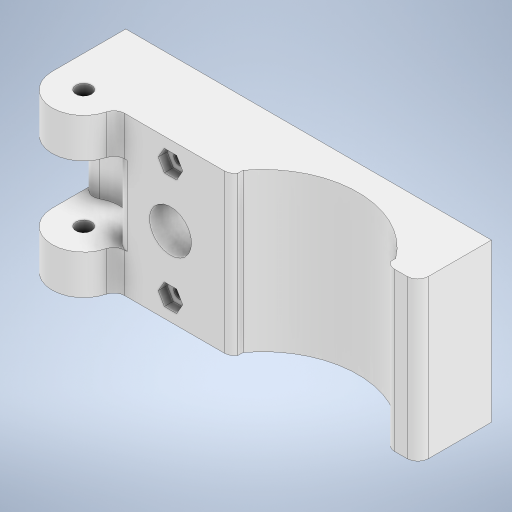
# Autodesk Inventor part: Bike_Mount_Right
Saved by Autodesk Inventor 2023 (Build 270158000, 158)
## iProperties
Created: 2023-01-23
Part Number: Bike_Mount_Right
Material: PC/ABS Plastic
Document SubType Name: Modeling
Designer: manny
Density: 0.357273 g/cm^3
Appearance: White
Author: manny
Autodesk Inventor part; units mm, degrees
ref_plane "YZ Plane" through (0, 0, 0) normal (1, 0, 0) x (0, 1, 0)
ref_plane "XZ Plane" through (0, 0, 0) normal (0, 1, 0) x (-1, 0, 0)
ref_plane "XY Plane" through (0, 0, 0) normal (0, 0, 1) x (1, 0, 0)
sketch "Sketch2" plane through (0, 0, 0) normal (0, 1, 0) x (-1, 0, 0)
  arc A0 (2, 14) -> (0, 12) centre (2, 12) ccw
  arc A1 (6.0742, 13.1179) -> (35.0957, 13.1179) centre (20.5849, 22.9) ccw
  line L0 (36.754, 14) -> (55.754, 14)
  arc A2 (69.5, 14) -> (57.6905, 15.5) centre (63.5, 14) ccw
  circle A3 centre (63.5, 14) radius 1.5
  arc A4 (55.754, 14) -> (57.6905, 15.5) centre (55.754, 16) ccw
  arc A5 (36.754, 14) -> (35.0957, 13.1179) centre (36.754, 12) ccw
  arc A6 (6.0742, 13.1179) -> (4.4158, 14) centre (4.4158, 12) ccw
  arc A7 (57.3882, 12.2181) -> (55.2287, 14) centre (55.2287, 11.8005) ccw
  line L1 (0, 12) -> (0, 0)
  line L2 (0, 0) -> (69.5, 0)
  line L3 (69.5, 14) -> (69.5, 0)
  arc A8 (57.3882, 12.2181) -> (69.5, 11.7415) centre (63.5, 13.4) ccw
  line L4 (4.4158, 14) -> (2, 14)
  point P0 (0, 0)
  point P1 (20.5849, 5.4)
  dimension "d3" = 2
  dimension "d17" = 3
  dimension "d18" = 2
  dimension "d137" = 2.1995
  dimension "d140" = 12
  dimension "d141" = 69.5
  dimension "d142" = 14
  dimension "d143" = 6
  dimension "d144" = 17.5
  dimension "d145" = 19
  dimension "d146" = 5.4
  dimension "d147" = 6.225
  dimension "d148" = 13.4
  constraints: 18 point on circle, 11 tangent, 10 end point, 9 centre point, 5 point on line, 3 horizontal, 2 vertical, 1 coincident, 1 equal radius, 1 horizontal alignment, 1 vertical alignment
  measures "d3" radius of A0
  measures "d17" diameter of A3
  measures "d18" radius of A4
  measures "d137" radius of A7
  measures "d140" distance from line of L2 A0.centre
  measures "d141" distance of L1.end L2.end
  measures "d142" distance of L3.start L2.end
  measures "d143" radius of A2
  measures "d144" radius of A1
  measures "d145" distance of L0.start L0.end
  measures "d146" distance from line of L2 point (20.585, 5.4)
  measures "d147" radius of A8
  measures "d148" vertical distance of point (0, 0) A8.centre
extrude "Extrusion1" add sketch "Sketch2" along normal mid plane 30
extrude "Extrusion2" cut sketch "Sketch2" along normal mid plane 15 contours A8 A7 L0 A4 A2 L3
sketch "Sketch7" plane through (0, -15, 0) normal (0, -1, 0) x (1, 0, 0)
  arc A0 (-4.4158, 14) -> (-6.0742, 13.1179) centre (-4.4158, 12) ccw projected
  line L0 (-6.0742, 13.1179) -> (-6.0742, 12.1179)
  arc A1 (-35.0957, 13.1179) -> (-6.0742, 13.1179) centre (-20.5849, 22.9) ccw projected
  line L1 (-35.0957, 13.1179) -> (-35.0957, 12.1179)
  arc A2 (-35.0957, 12.1179) -> (-6.0742, 12.1179) centre (-20.5849, 22.8831) ccw
  point P0 (0, 0)
  point P1 (-6.3389, 0)
  dimension "d59" = 1
  dimension "d60" = 1
  constraints: 4 end point, 2 point on circle, 2 vertical, 1 centre point
  measures "d59" distance of L0.start L0.end
  measures "d60" distance of L1.start L1.end
extrude "Extrusion10" cut sketch "Sketch7" against normal up to next
fillet "Fillet4" radius 2 1 edges at (-69.5, 0, 11.7415)
sketch "Sketch13" plane through (-55.754, -15, 14) normal (0, 0, 1) x (1, 0, 0)
  circle A0 centre (8.754, 15) radius 4
  line L0 (55.754, 0) -> (55.754, 30) projected
  line L1 (14.254, 18.1754) -> (14.254, 11.8246)
  line L2 (14.254, 11.8246) -> (8.754, 8.6491)
  line L3 (8.754, 8.6491) -> (3.254, 11.8246)
  line L4 (3.254, 11.8246) -> (3.254, 18.1754)
  line L5 (3.254, 18.1754) -> (8.754, 21.3509)
  line L6 (8.754, 21.3509) -> (14.254, 18.1754)
  line L7 (19, 0) -> (0, 0) projected
  circle A1 centre (8.754, 26) radius 1.1
  line L8 (8.754, 15) -> (25.6273, 15) construction
  line L9 (9.9232, 23.975) -> (7.5849, 23.975)
  line L10 (7.5849, 23.975) -> (6.4158, 26)
  line L11 (6.4158, 26) -> (7.5849, 28.025)
  line L12 (7.5849, 28.025) -> (9.9232, 28.025)
  line L13 (9.9232, 28.025) -> (11.0923, 26)
  line L14 (11.0923, 26) -> (9.9232, 23.975)
  circle A2 centre (8.754, 4) radius 1.1
  line L15 (9.9232, 6.025) -> (7.5849, 6.025)
  line L16 (7.5849, 6.025) -> (6.4158, 4)
  line L17 (6.4158, 4) -> (7.5849, 1.975)
  line L18 (7.5849, 1.975) -> (9.9232, 1.975)
  line L19 (9.9232, 1.975) -> (11.0923, 4)
  line L20 (11.0923, 4) -> (9.9232, 6.025)
  point P0 (55.754, 15)
  dimension "d99" = 8
  dimension "d106" = 47
  dimension "d131" = 11
  dimension "d132" = 15
  dimension "d159" = 2.2
  dimension "d160" = 11
  dimension "d163" = 4.05
  constraints: 38 end point, 9 symmetric about line, 5 coincident, 3 centre point, 2 horizontal, 1 vertical, 1 vertical alignment, 27 other
  measures "d99" diameter of A0
  measures "d106" distance of A0.centre point (55.754, 15)
  measures "d131" distance between parallel lines of L1 L4
  measures "d132" distance from line of A0.centre L7
  measures "d159" diameter of A1
  measures "d160" distance of A0.centre A1.centre
  measures "d163" distance between parallel lines of L9 L12
extrude "Extrusion15" cut sketch "Sketch13" against normal up to next contours A0
sketch "Sketch17" plane through (-55.754, -15, 14) normal (0, 0, 1) x (1, 0, 0)
  point P0 (55.754, 15)
sketch "Sketch19" plane through (0, 15, 0) normal (0, 0, -1) x (-1, 0, 0)
  circle A0 centre (47, -15) radius 4 projected
  line L0 (47, -21.4663) -> (41.4, -18.2332)
  line L1 (41.4, -18.2332) -> (41.4, -11.7668)
  line L2 (41.4, -11.7668) -> (47, -8.5337)
  line L3 (47, -8.5337) -> (52.6, -11.7668)
  line L4 (52.6, -11.7668) -> (52.6, -18.2332)
  line L5 (52.6, -18.2332) -> (47, -21.4663)
  point P0 (0, -15)
  dimension "d156" = 11.2
  constraints: 12 end point, 1 coincident, 1 vertical alignment, 13 other
  measures "d156" distance between parallel lines of L1 L4
extrude "Extrusion23" cut sketch "Sketch19" against normal blind 4.5
sketch "Sketch20" plane through (0, 15, 0) normal (0, 1, 0) x (1, 0, 0)
  point P0 (0, 0)
extrude "Extrusion24" cut sketch "Sketch13" against normal up to next contours A1 | A2
extrude "Extrusion25" cut sketch "Sketch13" against normal blind 1.7 contours A1 | L9 L10 L11 L12 L13 L14 | A2 | L20 L19 L18 L17 L16 L15
body "Solid1"
